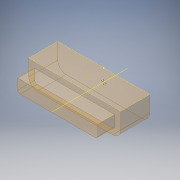
# Autodesk Inventor part: ps2conn
Saved by Autodesk Inventor 2019 (Build 230136000, 136)
## iProperties
Created: 2020-06-11
Part Number: ps2conn
Material: Generic
Document SubType Name: Modeling
Designer: assman
Density: 1 g/cm^3
Appearance: Oil
Author: assman
Autodesk Inventor part; units mm, degrees
ref_plane "YZ Plane" through (0, 0, 0) normal (1, 0, 0) x (0, 1, 0)
ref_plane "XZ Plane" through (0, 0, 0) normal (0, 1, 0) x (-1, 0, 0)
ref_plane "XY Plane" through (0, 0, 0) normal (0, 0, 1) x (1, 0, 0)
sketch "Sketch1" plane through (0, 0, 0) normal (0, 0, 1) x (1, 0, 0)
  line L0 (-22.25, 5.95) -> (22.25, 5.95) construction
  line L1 (22.25, 5.95) -> (22.25, -1.95)
  line L2 (18.25, -5.95) -> (-18.25, -5.95)
  line L3 (-22.25, -1.95) -> (-22.25, 5.95)
  line L4 (-22.25, 5.95) -> (22.25, -5.95) construction
  line L5 (22.25, 5.95) -> (-22.25, -5.95) construction
  arc A0 (-22.25, -1.95) -> (-18.25, -5.95) centre (-18.25, -1.95) ccw
  arc A1 (18.25, -5.95) -> (22.25, -1.95) centre (18.25, -1.95) ccw
  line L6 (-18.25, -5.95) -> (18.25, -5.95)
  line L7 (-22.25, -1.95) -> (-22.25, 5.95)
  line L8 (-22.25, 5.95) -> (22.25, 5.95)
  line L9 (22.25, 5.95) -> (22.25, -1.95)
  point P0 (0, 0)
  dimension "d0" = 44.5
  dimension "d1" = 11.9
  dimension "d2" = 4
  constraints: 20 end point, 5 point on line, 4 point on circle, 4 tangent, 2 centre point, 2 collinear, 2 midpoint, 2 parallel, 1 equal radius, 1 horizontal, 1 perpendicular
  measures "d0" distance of L4.end L5.end
  measures "d1" distance of L0.end L4.end
  measures "d2" radius of A0
extrude "Extrusion1" add sketch "Sketch1" along normal blind 14
sketch "Sketch2" plane through (0, 0, 14) normal (0, 0, 1) x (1, 0, 0)
  line L0 (-22.25, 5.95) -> (-22.25, -1.95) projected
  arc A0 (-22.25, -1.95) -> (-18.25, -5.95) centre (-18.25, -1.95) ccw projected
  line L1 (-18.25, -5.95) -> (18.25, -5.95) projected
  arc A1 (18.25, -5.95) -> (22.25, -1.95) centre (18.25, -1.95) ccw projected
  line L2 (22.25, -1.95) -> (22.25, 5.95) projected
  line L3 (22.25, 5.95) -> (-22.25, 5.95) projected
  line L4 (-19.3806, 3.0806) -> (-19.3806, -1.95)
  arc A2 (-19.3806, -1.95) -> (-18.25, -3.0806) centre (-18.25, -1.95) ccw
  line L5 (-18.25, -3.0806) -> (18.25, -3.0806)
  arc A3 (18.25, -3.0806) -> (19.3806, -1.95) centre (18.25, -1.95) ccw
  line L6 (19.3806, -1.95) -> (19.3806, 3.0806)
  line L7 (19.3806, 3.0806) -> (-19.3806, 3.0806)
  point P0 (0, 0)
  constraints: 8 end point, 4 point on circle, 2 centre point, 5 other
extrude "Extrusion2" add sketch "Sketch2" along normal blind 8.2 contours L7 L6 A3 L5 A2 L4
sketch "Sketch3" plane through (0, 0, 0) normal (0, 0, -1) x (-1, 0, 0)
  point P0 (0, 0)
  point P1 (0, 0)
  constraints: 1 coincident
sketch "Sketch4" plane through (-22.25, 5.95, 0) normal (0, 1, 0) x (1, 0, 0)
  line L0 (44.5, 0) -> (0, 0) construction
  line L1 (0, 0) -> (0, -14) construction
  line L2 (44.5, -14) -> (0, -14) construction
  line L3 (44.5, 0) -> (44.5, -14) construction
  point P0 (22.25, 0)
  point P1 (22.25, -7)
body "Solid1"
